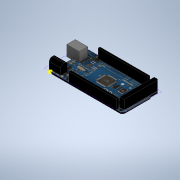
# Autodesk Inventor part: arduinomega
Saved by Autodesk Inventor 2021.5 (Build 255421000, 421)
## iProperties
Created: 2025-01-01
Part Number: arduinomega
Material: Generic
Document SubType Name: Modeling
Designer: email
Density: 1 g/cm^3
Appearance: Default
Author: email
Autodesk Inventor part; units mm, degrees
ref_plane "YZ Plane" through (0, 0, 0) normal (1, 0, 0) x (0, 1, 0)
ref_plane "XZ Plane" through (0, 0, 0) normal (0, 1, 0) x (-1, 0, 0)
ref_plane "XY Plane" through (0, 0, 0) normal (0, 0, 1) x (1, 0, 0)
sketch "Sketch1" plane through (0, 0, 0) normal (0, 1, 0) x (-1, 0, 0)
  line L0 (8.5074, -53.6851) -> (-102.7512, -53.6851) construction
  line L1 (-102.7512, -53.6851) -> (-102.7512, 0.3149) construction
  line L2 (-102.7512, 0.3149) -> (8.5074, 0.3149) construction
  line L3 (8.5074, 0.3149) -> (8.5074, -53.6851) construction
  line L4 (0, 0) -> (-101.6, 0)
  line L5 (-101.6, 0) -> (-101.6, -53.34)
  line L6 (-101.6, -53.34) -> (0, -53.34)
  line L7 (0, -53.34) -> (0, 0)
  circle A0 centre (-15.24, -50.8) radius 1.75
  circle A1 centre (-13.97, -2.54) radius 1.75
  circle A2 centre (-90.17, -50.8) radius 1.75
  circle A3 centre (-96.52, -2.54) radius 1.75
  line L8 (8.5074, -43.64) -> (-9, -43.64)
  line L9 (-9, -43.64) -> (-9, -31.74)
  line L10 (-9, -31.74) -> (8.5074, -31.74)
  line L11 (8.5074, -31.74) -> (8.5074, -43.64)
  line L12 (4.072, -12) -> (-12.22, -12)
  line L13 (-12.22, -12) -> (-12.22, -2.54)
  line L14 (-12.22, -2.54) -> (4.072, -2.54)
  line L15 (4.072, -2.54) -> (4.072, -12)
  line L16 (-26, -3) -> (-93, -3)
  line L17 (-93, -3) -> (-93, 0)
  line L18 (-93, 0) -> (-26, 0)
  line L19 (-26, 0) -> (-26, -3)
  line L20 (-93, -53.34) -> (-99, -53.34)
  line L21 (-99, -53.34) -> (-99, -5)
  line L22 (-99, -5) -> (-93, -5)
  line L23 (-93, -5) -> (-93, -53.34)
  line L24 (-18, -52) -> (-88, -52)
  line L25 (-88, -52) -> (-88, -49.3951)
  line L26 (-88, -49.3951) -> (-18, -49.3951)
  line L27 (-18, -49.3951) -> (-18, -52)
  line L28 (-97.4785, -53.34) -> (-100, -51.1451)
  line L29 (-100, -51.1451) -> (-100, -41)
  line L30 (-100, -41) -> (-101.6, -39)
  line L31 (-99.1411, 0) -> (-101.6, -2.8248)
  point P0 (-99, -52.0156)
  point P1 (-26, 0)
  dimension "d37" = 3.5
  dimension "d3" = 101.6
  dimension "d6" = 53.34
  dimension "d27" = 54
  dimension "d32" = 3.5
  dimension "d35" = 15.24
  dimension "d38" = 2.54
  dimension "d40" = 13.97
  dimension "d41" = 3.5
  dimension "d42" = 3.5
  dimension "d43" = 90.17
  dimension "d45" = 2.54
  dimension "d46" = 2.54
  dimension "d48" = 96.52
  dimension "d69" = 8.5074
  dimension "d70" = 9.7
  dimension "d71" = 11.9
  dimension "d73" = 2.54
  constraints: 56 end point, 12 parallel, 8 point on line, 6 horizontal, 6 perpendicular, 3 centre point, 1 horizontal alignment, 4 other
  measures "d3" distance of L5.end L6.end
  measures "d6" distance of L4.end L5.end
  measures "d27" distance of L2.end L0.start
  measures "d32" diameter of A0
  measures "d35" distance from line of L7 A0.centre
  measures "d38" distance from line of L4 point (-13.97, -2.54)
  measures "d40" distance from line of L7 point (-13.97, -2.54)
  measures "d41" diameter of A2
  measures "d42" diameter of A3
  measures "d43" distance from line of L7 A2.centre
  measures "d45" distance from line of L6 A2.centre
  measures "d46" distance from line of L4 A3.centre
  measures "d48" distance from line of L7 A3.centre
  measures "d69" distance between parallel lines of L7 L3
  measures "d70" distance between parallel lines of L6 L8
  measures "d71" distance between parallel lines of L10 L8
  measures "d73" distance from line of L6 A0.centre
extrude "Extrusion1" add sketch "Sketch1" along normal blind 2 contours L7 L14 L13 L12 L10 L9 L8 L6 L23 L22 L21 L28 L29 L30 L5 L31 L4 L17 L16 L19 | L19 L16 L17 L4 | L7 L12 L13 L14 | L7 L8 L9 L10 | L6 L28 L21 L22 L23 | L24 L25 L26 L27
sketch "Sketch2" plane through (0, 2, 0) normal (0, 1, 0) x (1, 0, 0)
  line L0 (-8.4913, 53.8189) -> (102.7673, 53.8189) construction
  line L1 (102.7673, 53.8189) -> (102.7673, -0.1811) construction
  line L2 (102.7673, -0.1811) -> (-8.4913, -0.1811) construction
  line L3 (-8.4913, -0.1811) -> (-8.4913, 53.8189) construction
  point P0 (0, 0)
  dimension "d60" = 54
  constraints: 2 other
  measures "d60" distance of L0.end L1.end
extrude "Extrusion2" add sketch "Sketch1" along normal blind 15 contours L19 L16 L17 L4 | L14 L15 L12 L7 | L7 L12 L13 L14 | L10 L11 L8 L7 | L7 L8 L9 L10 | L6 L28 L21 L22 L23 | L24 L25 L26 L27
fillet "Fillet1" radius 4 2 edges at (4.074, 15, -2.54) (4.074, 15, -12)
body "Solid1"
